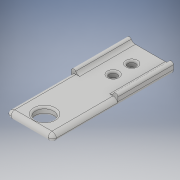
# Autodesk Inventor part: Side Attatchment
Saved by Autodesk Inventor 2019 (Build 230136000, 136)
## iProperties
Created: 2019-01-05
Part Number: Side Attatchment
Material: Generic
Document SubType Name: Modeling
Designer: ashle
Density: 1 g/cm^3
Appearance: Default
Author: ashle
Autodesk Inventor part; units mm, degrees
ref_plane "YZ Plane" through (0, 0, 0) normal (1, 0, 0) x (0, 1, 0)
ref_plane "XZ Plane" through (0, 0, 0) normal (0, 1, 0) x (-1, 0, 0)
ref_plane "XY Plane" through (0, 0, 0) normal (0, 0, 1) x (1, 0, 0)
sketch "Sketch2" plane through (0, 0, 0) normal (0, 1, 0) x (-1, 0, 0)
  line L0 (12.5, 32.5) -> (-12.5, 32.5)
  line L1 (-12.5, 32.5) -> (-12.5, -32.5)
  line L2 (-12.5, -32.5) -> (12.5, -32.5)
  line L3 (12.5, -32.5) -> (12.5, 32.5)
  line L4 (0, 0) -> (0, -32.5) construction
  line L5 (0, 0) -> (0, 32.5) construction
  line L6 (0, 0) -> (12.5, 0) construction
  line L7 (0, 0) -> (-12.5, 0) construction
  dimension "d45" = 25
  dimension "d46" = 65
  constraints: 16 end point, 4 midpoint, 2 collinear, 2 parallel, 1 horizontal, 1 perpendicular
  measures "d45" distance of L0.start L0.end
  measures "d46" distance of L2.end L0.start
extrude "Main Body Sketch" add sketch "Sketch2" along normal blind 6
sketch "Sketch3" plane through (0, 6, 0) normal (0, 1, 0) x (1, 0, 0)
  line L0 (10.5, 2.5) -> (10.5, 32.5)
  line L1 (10.5, 32.5) -> (-10.5, 32.5)
  line L2 (-10.5, 32.5) -> (-10.5, 2.5)
  line L3 (12.5, 32.5) -> (-12.5, 32.5) projected
  line L4 (-12.5, -32.5) -> (12.5, -32.5) projected
  line L5 (-12.5, 32.5) -> (-12.5, -32.5) projected
  line L6 (12.5, -32.5) -> (12.5, 32.5) projected
  line L7 (12.5, -32.5) -> (-12.5, -32.5)
  line L8 (-12.5, -32.5) -> (-12.5, 2.5)
  line L9 (12.5, 2.5) -> (12.5, -32.5)
  line L10 (-12.5, 2.5) -> (-10.5, 2.5)
  line L11 (10.5, 2.5) -> (12.5, 2.5)
  point P0 (0, 0)
  dimension "d51" = 2
  dimension "d52" = 2
  dimension "d61" = 30
  dimension "d62" = 30
  constraints: 16 end point, 4 collinear, 4 parallel, 1 horizontal, 1 perpendicular
  measures "d51" distance between parallel lines of L5 L2
  measures "d52" distance between parallel lines of L6 L0
  measures "d61" distance between parallel lines of L3 L10
  measures "d62" distance between parallel lines of L3 L11
extrude "Edges Cut" cut sketch "Sketch3" against normal blind 2 contours L11 L6 L4 L5 L10 L2 L1 L0
sketch "Sketch4" plane through (0, 4, 0) normal (0, 1, 0) x (1, 0, 0)
  circle A0 centre (0, -24.5) radius 4.8537
  line L0 (-10.5, 32.5) -> (10.5, 32.5) projected
  line L1 (12.5, -32.5) -> (-12.5, -32.5) projected
  line L2 (-12.5, -32.5) -> (-12.5, 2.5) projected
  circle A1 centre (0, 12.5) radius 2.15
  circle A2 centre (0, 22.5) radius 2.15
  line L3 (-10.5, 2.5) -> (-10.5, 32.5) projected
  line L4 (10.5, 32.5) -> (10.5, 2.5) projected
  line L5 (12.5, 2.5) -> (12.5, -32.5) projected
  point P0 (0, 0)
  dimension "d63" = 57
  dimension "d64" = 8
  dimension "d66" = 12.5
  dimension "d73" = 4.3
  dimension "d74" = 4.3
  dimension "d75" = 10.5
  dimension "d76" = 21
  dimension "d77" = 10.5
  dimension "d78" = 10
  dimension "d79" = 10
  dimension "d80" = 25
  constraints: 3 centre point
  measures "d63" distance from line of A0.centre L0
  measures "d64" distance from line of L1 A0.centre
  measures "d66" distance from line of L2 A0.centre
  measures "d73" diameter of A1
  measures "d74" diameter of A2
  measures "d75" distance from line of L3 A1.centre
  measures "d76" distance between parallel lines of L3 L4
  measures "d77" distance from line of L3 A2.centre
  measures "d78" distance from line of L0 A2.centre
  measures "d79" distance of A2.centre A1.centre
  measures "d80" distance between parallel lines of L2 L5
extrude "Holes Cuts" cut sketch "Sketch4" against normal up to surface (4 mm away)
fillet "Fillet5" radius 2.5 6 edges at (-10.5, 4, -17.5) (10.5, 4, -17.5) (12.5, 4, 15) (-12.5, 4, 15) (12.5, 0, 0) (-12.5, 0, 0)
fillet "Fillet6" radius 1.2 4 edges at (-10.5, 6, -17.5) (-12.5, 6, -17.5) (10.5, 6, -17.5) (12.5, 6, -17.5)
fillet "Fillet7" radius 2 2 edges at (0, 0, 32.5) (0, 4, 32.5)
fillet "Fillet9" radius 1 6 edges at (-4.8537, 4, 24.5) (-4.8537, 0, 24.5) (-2.15, 4, -12.5) (-2.15, 4, -22.5) (-2.15, 0, -12.5) (-2.15, 0, -22.5)
equation "\"d46\" = AH"
equation "\"d61\" = TMROL"
equation "\"d62\" = TMROL"
equation "\"d63\" = -uw + AH - 0.5 * BD"
equation "\"d66\" = 0.5 * d80"
equation "\"d73\" = sut"
equation "\"d74\" = sut"
equation "\"d75\" = 0.5 * d76"
equation "\"d77\" = d75"
equation "\"d78\" = BSHH"
equation "\"d79\" = BSHH"
equation "\"AH\" = 65"
equation "\"BD\" = 4"
equation "\"TMROL\" = 30"
equation "\"uw\" = 6"
equation "\"sut\" = 4.3"
equation "\"BSHH\" = 10"
body "Solid1"
